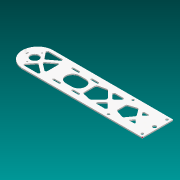
# Autodesk Inventor part: bovenarm - rechts
Saved by Autodesk Inventor 2020 (Build 240168000, 168)
## iProperties
Created: 2020-05-18
Part Number: bovenarm - rechts
Material: Aluminum 6061
Document SubType Name: Modeling
Designer: stefa
Density: 2.7 g/cm^3
Appearance: Aluminum - Polished
Mass: 90.489 g
Surface Area: 217.27 cm^2
Volume: 33.5144 cm^3
Author: stefa
Autodesk Inventor part; units mm, degrees
ref_plane "YZ Plane" through (0, 0, 0) normal (1, 0, 0) x (0, 1, 0)
ref_plane "XZ Plane" through (0, 0, 0) normal (0, 1, 0) x (-1, 0, 0)
ref_plane "XY Plane" through (0, 0, 0) normal (0, 0, 1) x (1, 0, 0)
sketch "Sketch1" plane through (0, 0, 0) normal (0, 1, 0) x (-1, 0, 0)
  line L0 (0, 0) -> (220, 0)
  line L1 (220, 0) -> (220, -50)
  line L2 (220, -50) -> (0, -50)
  line L3 (0, -50) -> (0, 0)
  circle A0 centre (200, -25) radius 7
  line L4 (138.262, -25) -> (128.262, -25) construction
  line L5 (138.262, -13.9) -> (128.262, -13.9)
  line L6 (128.262, -36.1) -> (138.262, -36.1)
  arc A1 (138.262, -36.1) -> (138.262, -13.9) centre (138.262, -25) ccw
  arc A2 (128.262, -13.9) -> (128.262, -36.1) centre (128.262, -25) ccw
  line L7 (153.762, -40.5) -> (143.762, -40.5) construction
  line L8 (153.762, -38.95) -> (143.762, -38.95)
  line L9 (143.762, -42.05) -> (153.762, -42.05)
  arc A3 (153.762, -42.05) -> (153.762, -38.95) centre (153.762, -40.5) ccw
  arc A4 (143.762, -38.95) -> (143.762, -42.05) centre (143.762, -40.5) ccw
  line L10 (112.762, -42.05) -> (122.762, -42.05)
  arc A5 (122.762, -42.05) -> (122.762, -38.95) centre (122.762, -40.5) ccw
  line L11 (122.762, -40.5) -> (112.762, -40.5) construction
  line L12 (122.762, -38.95) -> (112.762, -38.95)
  arc A6 (112.762, -38.95) -> (112.762, -42.05) centre (112.762, -40.5) ccw
  line L13 (143.762, -11.05) -> (153.762, -11.05)
  arc A7 (153.762, -11.05) -> (153.762, -7.95) centre (153.762, -9.5) ccw
  line L14 (153.762, -9.5) -> (143.762, -9.5) construction
  line L15 (153.762, -7.95) -> (143.762, -7.95)
  arc A8 (143.762, -7.95) -> (143.762, -11.05) centre (143.762, -9.5) ccw
  line L16 (112.762, -11.05) -> (122.762, -11.05)
  arc A9 (122.762, -11.05) -> (122.762, -7.95) centre (122.762, -9.5) ccw
  line L17 (122.762, -9.5) -> (112.762, -9.5) construction
  line L18 (122.762, -7.95) -> (112.762, -7.95)
  arc A10 (112.762, -7.95) -> (112.762, -11.05) centre (112.762, -9.5) ccw
  circle A11 centre (160, -45) radius 2.05
  circle A12 centre (160, -5) radius 2.05
  circle A13 centre (60, -45) radius 2.05
  circle A14 centre (60, -5) radius 2.05
  circle A15 centre (5, -25) radius 3
  circle A16 centre (5, -5) radius 2.05
  circle A17 centre (5, -45) radius 2.05
  line L19 (220, -25) -> (171.1069, -25) construction
  line L20 (199, -36) -> (201, -36)
  line L21 (201, -36) -> (201, -38)
  line L22 (201, -38) -> (199, -38)
  line L23 (199, -38) -> (199, -36)
  line L24 (199, -36) -> (201, -38) construction
  line L25 (201, -36) -> (199, -38) construction
  line L26 (213, -23) -> (211, -23)
  line L27 (211, -23) -> (211, -27)
  line L28 (211, -27) -> (213, -27)
  line L29 (213, -27) -> (213, -23)
  line L30 (213, -23) -> (211, -27) construction
  line L31 (211, -23) -> (213, -27) construction
  line L32 (199, -14) -> (201, -14)
  line L33 (201, -14) -> (201, -12)
  line L34 (201, -12) -> (199, -12)
  line L35 (199, -12) -> (199, -14)
  line L36 (199, -14) -> (201, -12) construction
  line L37 (201, -14) -> (199, -12) construction
  point P0 (133.262, -25)
  point P1 (148.762, -40.5)
  point P2 (117.762, -40.5)
  point P3 (148.762, -9.5)
  point P4 (117.762, -9.5)
  point P5 (0, -25)
  point P6 (200, -37)
  point P7 (200, -37)
  point P8 (212, -25)
  point P9 (200, -13)
  point P10 (200, -13)
  dimension "d0" = 220
  dimension "d1" = 50
  dimension "d16" = 14
  dimension "d18" = 25
  dimension "d24" = 22.2
  dimension "d25" = 3.1
  dimension "d26" = 10
  dimension "d27" = 10
  dimension "d28" = 66.738
  dimension "d29" = 25
  dimension "d31" = 15.5
  dimension "d32" = 15.5
  dimension "d35" = 31
  dimension "d38" = 31
  dimension "d42" = 4.1
  dimension "d44" = 5
  dimension "d47" = 40
  dimension "d50" = 100
  dimension "d53" = 6
  dimension "d56" = 5
  dimension "d58" = 20
  dimension "d59" = 20
  dimension "d86" = 160
  dimension "d87" = 200
  dimension "d95" = 2
  dimension "d96" = 2
  dimension "d97" = 12
  dimension "d98" = 2
  dimension "d99" = 4
  dimension "d100" = 12
  dimension "d101" = 4.1
  constraints: 86 end point, 20 point on circle, 18 centre point, 11 midpoint, 9 parallel, 8 tangent, 7 horizontal, 6 symmetric about line, 3 perpendicular, 3 vertical alignment, 2 vertical, 1 equal radius, 1 horizontal alignment, 1 point on line, 42 other
  measures "d0" distance of L1.end L2.end
  measures "d1" distance of L0.end L1.end
  measures "d16" diameter of A0
  measures "d18" distance from line of L0 A0.centre
  measures "d24" diameter of A2
  measures "d25" diameter of A4
  measures "d26" distance of L9.start L9.end
  measures "d27" distance of L6.start L6.end
  measures "d28" distance of A0.centre point (133.262, -25)
  measures "d29" distance from line of L0 point (133.262, -25)
  measures "d31" horizontal distance of point (133.262, -25) point (148.762, -40.5)
  measures "d32" horizontal distance of point (148.762, -40.5) point (133.262, -25)
  measures "d35" distance of L9.start L10.start
  measures "d38" distance of L9.start L13.start
  measures "d42" diameter of A11
  measures "d44" distance from line of A11.centre L2
  measures "d47" distance of A11.centre A12.centre
  measures "d50" distance of A11.centre A13.centre
  measures "d53" diameter of A15
  measures "d56" distance from line of L3 A15.centre
  measures "d58" distance of A16.centre A15.centre
  measures "d59" distance of A17.centre A15.centre
  measures "d86" distance from line of L3 A11.centre
  measures "d87" distance from line of L3 A0.centre
  measures "d95" distance of L21.end L22.end
  measures "d96" distance of L20.end L21.end
  measures "d97" distance of A0.centre point (200, -37)
  measures "d98" distance of L28.end L27.end
  measures "d99" distance of L26.end L27.end
  measures "d100" distance of A0.centre point (212, -25)
  measures "d101" diameter of A16
extrude "Extrusion1" add sketch "Sketch1" along normal blind 2 contours L0 L1 L2 L3 | A11 | A12
fillet "Fillet1" radius 25 2 edges at (-220, 1, 0) (-220, 1, -50)
sketch "Sketch7" plane through (0, 2, 0) normal (0, 1, 0) x (1, 0, 0)
  point P0 (0, 0)
sketch "Sketch8" plane through (0, 2, 0) normal (0, 1, 0) x (1, 0, 0)
  arc A0 (-143.762, 38.95) -> (-143.762, 42.05) centre (-143.762, 40.5) ccw projected
  line L0 (-143.762, 38.95) -> (-153.762, 38.95) projected
  arc A1 (-153.762, 42.05) -> (-153.762, 38.95) centre (-153.762, 40.5) ccw projected
  line L1 (-153.762, 42.05) -> (-143.762, 42.05) projected
  line L2 (-122.762, 42.05) -> (-112.762, 42.05) projected
  arc A2 (-112.762, 38.95) -> (-112.762, 42.05) centre (-112.762, 40.5) ccw projected
  line L3 (-112.762, 38.95) -> (-122.762, 38.95) projected
  arc A3 (-122.762, 42.05) -> (-122.762, 38.95) centre (-122.762, 40.5) ccw projected
  line L4 (-153.762, 11.05) -> (-143.762, 11.05) projected
  arc A4 (-143.762, 7.95) -> (-143.762, 11.05) centre (-143.762, 9.5) ccw projected
  line L5 (-143.762, 7.95) -> (-153.762, 7.95) projected
  arc A5 (-153.762, 11.05) -> (-153.762, 7.95) centre (-153.762, 9.5) ccw projected
  line L6 (-128.262, 13.9) -> (-138.262, 13.9) projected
  arc A6 (-138.262, 36.1) -> (-138.262, 13.9) centre (-138.262, 25) ccw projected
  line L7 (-138.262, 36.1) -> (-128.262, 36.1) projected
  arc A7 (-128.262, 13.9) -> (-128.262, 36.1) centre (-128.262, 25) ccw projected
  line L8 (-122.762, 11.05) -> (-112.762, 11.05) projected
  arc A8 (-112.762, 7.95) -> (-112.762, 11.05) centre (-112.762, 9.5) ccw projected
  line L9 (-112.762, 7.95) -> (-122.762, 7.95) projected
  arc A9 (-122.762, 11.05) -> (-122.762, 7.95) centre (-122.762, 9.5) ccw projected
  circle A10 centre (-200, 25) radius 7 projected
  circle A11 centre (-60, 45) radius 2.05 projected
  circle A12 centre (-60, 5) radius 2.05 projected
  circle A13 centre (-5, 25) radius 3 projected
  circle A14 centre (-5, 5) radius 2.05 projected
  circle A15 centre (-5, 45) radius 2.05 projected
  arc A16 (-195, 50) -> (-195, 0) centre (-195, 25) ccw projected
  line L10 (-195, 0) -> (0, 0) projected
  line L11 (0, 0) -> (0, 50) projected
  line L12 (0, 50) -> (-195, 50) projected
  line L13 (-30.9142, 20) -> (-24, 13)
  line L14 (-24, 13) -> (-36, 13)
  line L15 (-36, 13) -> (-30.9142, 20)
  line L16 (-34.3896, 25) -> (-43.7942, 12.0557)
  line L17 (-43.7942, 12.0557) -> (-59.0111, 17)
  line L18 (-59.0111, 17) -> (-59.0111, 33)
  line L19 (-59.0111, 33) -> (-43.7942, 37.9443)
  line L20 (-43.7942, 37.9443) -> (-34.3896, 25)
  line L21 (-5, 25) -> (-200, 25) construction
  line L22 (0, 0) -> (0, 50) construction
  line L23 (-30.9142, 30) -> (-24, 37)
  line L24 (-24, 37) -> (-36, 37)
  line L25 (-36, 37) -> (-30.9142, 30)
  line L26 (-64.0111, 25) -> (-64.0111, 15)
  line L27 (-64.0111, 15) -> (-74.0111, 25)
  line L28 (-77.5111, 21.4289) -> (-89.0111, 9.9289)
  line L29 (-89.0111, 9.9289) -> (-66.0111, 9.9289)
  line L30 (-66.0111, 9.9289) -> (-77.5111, 21.4289)
  line L31 (-195, 0) -> (0, 0) projected
  line L32 (-64.0111, 25) -> (-64.0111, 35)
  line L33 (-64.0111, 35) -> (-74.0111, 25)
  line L34 (-77.5111, 28.5711) -> (-89.0111, 40.0711)
  line L35 (-89.0111, 40.0711) -> (-66.0111, 40.0711)
  line L36 (-66.0111, 40.0711) -> (-77.5111, 28.5711)
  line L37 (-81.0111, 25) -> (-95.5108, 10.5003)
  line L38 (-95.5108, 10.5003) -> (-111.0111, 14)
  line L39 (-111.0111, 14) -> (-111.0111, 25)
  line L40 (-81.0111, 25) -> (-95.5108, 39.4997)
  line L41 (-95.5108, 39.4997) -> (-111.0111, 36)
  line L42 (-111.0111, 36) -> (-111.0111, 25)
  line L43 (-170.262, 25) -> (-170.262, 38)
  line L44 (-170.262, 38) -> (-187.262, 25)
  line L45 (-170.262, 25) -> (-170.262, 12)
  line L46 (-170.262, 12) -> (-187.262, 25)
  point P0 (-48, 25)
  dimension "d60" = 12
  dimension "d61" = 7
  dimension "d62" = 16
  dimension "d63" = 48
  dimension "d64" = 24
  dimension "d65" = 5
  dimension "d66" = 5
  dimension "d67" = 45
  dimension "d68" = 10
  dimension "d69" = 23
  dimension "d70" = 7
  dimension "d71" = 5
  dimension "d72" = 5
  dimension "d73" = 11
  dimension "d74" = 30
  dimension "d75" = 15.5003
  dimension "d76" = 13
  dimension "d77" = 17
  dimension "d78" = 32
  constraints: 64 end point, 10 vertical alignment, 5 parallel, 3 vertical, 2 horizontal, 1 perpendicular, 21 other
  measures "d60" distance of L13.end L14.end
  measures "d61" distance from line of L14 L13.start
  measures "d62" distance of L17.end L18.end
  measures "d63" distance from line of L11 point (-48, 25)
  measures "d64" distance from line of L11 L13.end
  measures "d66" distance between parallel lines of L18 L26
  measures "d67" angle of L26 L27
  measures "d68" distance of L26.start L26.end
  measures "d69" distance of L28.end L29.end
  measures "d70" horizontal distance of L17.end L29.end
  measures "d71" distance between parallel lines of L30 L27
  measures "d72" distance between parallel lines of L28 L37
  measures "d73" distance of L38.end L39.end
  measures "d74" distance of L37.start L39.end
  measures "d75" horizontal distance of L37.end L38.end
  measures "d76" distance of L43.start L43.end
  measures "d77" distance of L43.start L44.end
  measures "d78" distance of A6.centre L43.start
extrude "Extrusion2" cut sketch "Sketch8" against normal blind 10 contours L13 L14 L15 | L16 L17 L18 L19 L20 | L25 L24 L23 | L30 L29 L28 | L34 L35 L36 | L37 L38 L39 L42 L41 L40 | L45 L46 L44 L43
fillet "Fillet2" radius 2 3 edges at (-187.262, 1, -25) (-170.262, 1, -38) (-170.262, 1, -12)
fillet "Fillet3" radius 3 5 edges at (-111.0111, 1, -36) (-95.5108, 1, -39.4997) (-81.0111, 1, -25) (-95.5108, 1, -10.5003) (-111.0111, 1, -14)
fillet "Fillet4" radius 2 6 edges at (-89.0111, 1, -40.0711) (-66.0111, 1, -40.0711) (-77.5111, 1, -28.5711) (-89.0111, 1, -9.9289) (-77.5111, 1, -21.4289) (-66.0111, 1, -9.9289)
fillet "Fillet5" radius 2 5 edges at (-43.7942, 1, -37.9443) (-59.0111, 1, -33) (-59.0111, 1, -17) (-43.7942, 1, -12.0557) (-34.3896, 1, -25)
fillet "Fillet6" radius 1 6 edges at (-24, 1, -37) (-36, 1, -37) (-30.9142, 1, -20) (-30.9142, 1, -30) (-24, 1, -13) (-36, 1, -13)
sketch "Sketch9" plane through (0, 2, 0) normal (0, 1, 0) x (1, 0, 0)
  line L0 (-78.9253, 29.9853) -> (-85.5968, 36.6569) projected
  arc A0 (-84.1826, 40.0711) -> (-85.5968, 36.6569) centre (-84.1826, 38.0711) ccw projected
  line L1 (-84.1826, 40.0711) -> (-70.8395, 40.0711) projected
  arc A1 (-69.4253, 36.6569) -> (-70.8395, 40.0711) centre (-70.8395, 38.0711) ccw projected
  line L2 (-69.4253, 36.6569) -> (-76.0968, 29.9853) projected
  arc A2 (-78.9253, 29.9853) -> (-76.0968, 29.9853) centre (-77.5111, 31.3995) ccw projected
  line L3 (-34.8464, 14.5878) -> (-31.6067, 19.0468) projected
  arc A3 (-30.0863, 19.1618) -> (-31.6067, 19.0468) centre (-30.7977, 18.459) ccw projected
  line L4 (-30.0863, 19.1618) -> (-25.6819, 14.7027) projected
  arc A4 (-26.3933, 13) -> (-25.6819, 14.7027) centre (-26.3933, 14) ccw projected
  line L5 (-26.3933, 13) -> (-34.0374, 13) projected
  arc A5 (-34.8464, 14.5878) -> (-34.0374, 13) centre (-34.0374, 14) ccw projected
  line L6 (-76.0968, 20.0147) -> (-69.4253, 13.3431) projected
  arc A6 (-70.8395, 9.9289) -> (-69.4253, 13.3431) centre (-70.8395, 11.9289) ccw projected
  line L7 (-70.8395, 9.9289) -> (-84.1826, 9.9289) projected
  arc A7 (-85.5968, 13.3431) -> (-84.1826, 9.9289) centre (-84.1826, 11.9289) ccw projected
  line L8 (-85.5968, 13.3431) -> (-78.9253, 20.0147) projected
  arc A8 (-76.0968, 20.0147) -> (-78.9253, 20.0147) centre (-77.5111, 18.6005) ccw projected
  line L9 (-83.1324, 22.8787) -> (-94.3416, 11.6695) projected
  arc A9 (-97.1236, 10.8645) -> (-94.3416, 11.6695) centre (-96.4629, 13.7908) ccw projected
  line L10 (-97.1236, 10.8645) -> (-108.6718, 13.4718) projected
  arc A10 (-111.0111, 16.3982) -> (-108.6718, 13.4718) centre (-108.0111, 16.3982) ccw projected
  line L11 (-111.0111, 16.3982) -> (-111.0111, 33.6018) projected
  arc A11 (-108.6718, 36.5282) -> (-111.0111, 33.6018) centre (-108.0111, 33.6018) ccw projected
  line L12 (-108.6718, 36.5282) -> (-97.1236, 39.1355) projected
  arc A12 (-94.3416, 38.3305) -> (-97.1236, 39.1355) centre (-96.4629, 36.2092) ccw projected
  line L13 (-94.3416, 38.3305) -> (-83.1324, 27.1213) projected
  arc A13 (-83.1324, 22.8787) -> (-83.1324, 27.1213) centre (-85.2537, 25) ccw projected
  line L14 (-25.6819, 35.2973) -> (-30.0863, 30.8382) projected
  arc A14 (-31.6067, 30.9532) -> (-30.0863, 30.8382) centre (-30.7977, 31.541) ccw projected
  line L15 (-31.6067, 30.9532) -> (-34.8464, 35.4122) projected
  arc A15 (-34.0374, 37) -> (-34.8464, 35.4122) centre (-34.0374, 36) ccw projected
  line L16 (-34.0374, 37) -> (-26.3933, 37) projected
  arc A16 (-25.6819, 35.2973) -> (-26.3933, 37) centre (-26.3933, 36) ccw projected
  line L17 (-57.6291, 33.449) -> (-45.1761, 37.4952) projected
  arc A17 (-42.94, 36.7687) -> (-45.1761, 37.4952) centre (-44.5581, 35.5931) ccw projected
  line L18 (-42.94, 36.7687) -> (-35.2437, 26.1756) projected
  arc A18 (-35.2437, 23.8244) -> (-35.2437, 26.1756) centre (-36.8617, 25) ccw projected
  line L19 (-35.2437, 23.8244) -> (-42.94, 13.2313) projected
  arc A19 (-45.1761, 12.5048) -> (-42.94, 13.2313) centre (-44.5581, 14.4069) ccw projected
  line L20 (-45.1761, 12.5048) -> (-57.6291, 16.551) projected
  arc A20 (-59.0111, 18.4531) -> (-57.6291, 16.551) centre (-57.0111, 18.4531) ccw projected
  line L21 (-59.0111, 18.4531) -> (-59.0111, 31.5469) projected
  arc A21 (-57.6291, 33.449) -> (-59.0111, 31.5469) centre (-57.0111, 31.5469) ccw projected
  line L22 (-173.4769, 14.4585) -> (-185.1844, 23.4113) projected
  arc A22 (-185.1844, 26.5887) -> (-185.1844, 23.4113) centre (-183.9695, 25) ccw projected
  line L23 (-185.1844, 26.5887) -> (-173.4769, 35.5415) projected
  arc A23 (-170.262, 33.9528) -> (-173.4769, 35.5415) centre (-172.262, 33.9528) ccw projected
  line L24 (-170.262, 33.9528) -> (-170.262, 16.0472) projected
  arc A24 (-173.4769, 14.4585) -> (-170.262, 16.0472) centre (-172.262, 16.0472) ccw projected
  arc A25 (-195, 50) -> (-195, 0) centre (-195, 25) ccw projected
  line L25 (-195, 0) -> (0, 0) projected
  line L26 (0, 0) -> (0, 50) projected
  line L27 (0, 50) -> (-195, 50) projected
  circle A26 centre (-5, 45) radius 2.05 projected
  circle A27 centre (-5, 5) radius 2.05 projected
  circle A28 centre (-5, 25) radius 3 projected
  circle A29 centre (-60, 5) radius 2.05 projected
  circle A30 centre (-60, 45) radius 2.05 projected
  circle A31 centre (-200, 25) radius 7 projected
  arc A32 (-112.762, 7.95) -> (-112.762, 11.05) centre (-112.762, 9.5) ccw projected
  line L28 (-112.762, 7.95) -> (-122.762, 7.95) projected
  arc A33 (-122.762, 11.05) -> (-122.762, 7.95) centre (-122.762, 9.5) ccw projected
  line L29 (-122.762, 11.05) -> (-112.762, 11.05) projected
  line L30 (-138.262, 36.1) -> (-128.262, 36.1) projected
  arc A34 (-128.262, 13.9) -> (-128.262, 36.1) centre (-128.262, 25) ccw projected
  line L31 (-128.262, 13.9) -> (-138.262, 13.9) projected
  arc A35 (-138.262, 36.1) -> (-138.262, 13.9) centre (-138.262, 25) ccw projected
  arc A36 (-143.762, 7.95) -> (-143.762, 11.05) centre (-143.762, 9.5) ccw projected
  line L32 (-143.762, 7.95) -> (-153.762, 7.95) projected
  arc A37 (-153.762, 11.05) -> (-153.762, 7.95) centre (-153.762, 9.5) ccw projected
  line L33 (-153.762, 11.05) -> (-143.762, 11.05) projected
  line L34 (-112.762, 38.95) -> (-122.762, 38.95) projected
  arc A38 (-122.762, 42.05) -> (-122.762, 38.95) centre (-122.762, 40.5) ccw projected
  line L35 (-122.762, 42.05) -> (-112.762, 42.05) projected
  arc A39 (-112.762, 38.95) -> (-112.762, 42.05) centre (-112.762, 40.5) ccw projected
  line L36 (-143.762, 38.95) -> (-153.762, 38.95) projected
  arc A40 (-153.762, 42.05) -> (-153.762, 38.95) centre (-153.762, 40.5) ccw projected
  line L37 (-153.762, 42.05) -> (-143.762, 42.05) projected
  arc A41 (-143.762, 38.95) -> (-143.762, 42.05) centre (-143.762, 40.5) ccw projected
  line L38 (-189.1982, 20.1863) -> (-201.3393, 5)
  line L39 (-201.3393, 5) -> (-169.3393, 5)
  line L40 (-169.3393, 5) -> (-189.1982, 20.1863)
  line L41 (-173.4769, 14.4585) -> (-185.1844, 23.4113) projected
  line L42 (-195, 0) -> (0, 0) projected
  line L43 (-200, 25) -> (-5, 25) construction
  line L44 (-189.1982, 29.8137) -> (-201.3393, 45)
  line L45 (-201.3393, 45) -> (-169.3393, 45)
  line L46 (-169.3393, 45) -> (-189.1982, 29.8137)
  dimension "d88" = 25
  dimension "d89" = 5
  dimension "d90" = 5
  dimension "d91" = 32
  constraints: 14 end point, 3 symmetric about line, 2 horizontal, 2 parallel
  measures "d88" distance of L39.end L38.start
  measures "d89" distance between parallel lines of L22 L40
  measures "d90" distance between parallel lines of L25 L39
  measures "d91" distance of L38.end L39.end
extrude "Extrusion3" cut sketch "Sketch9" against normal blind 10 contours L40 L39 L38 | L44 L45 L46
fillet "Fillet7" radius 2 6 edges at (-201.3393, 1, -45) (-169.3393, 1, -45) (-189.1982, 1, -29.8137) (-189.1982, 1, -20.1863) (-169.3393, 1, -5) (-201.3393, 1, -5)
equation "\"d18\" = 0.5 * d1"
equation "\"d59\" = d58"
body "Solid1"
